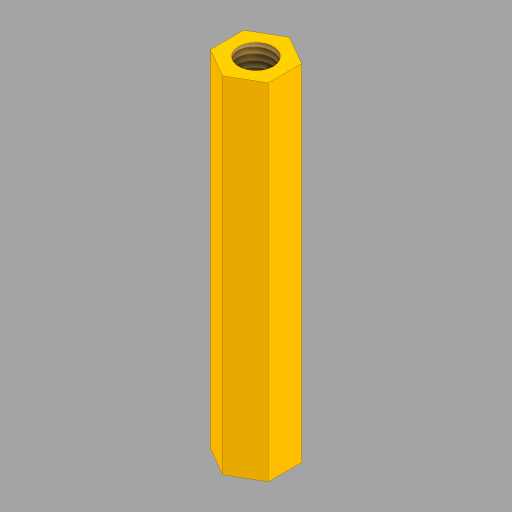
# Autodesk Inventor part: stoyka_40mm
Saved by Autodesk Inventor 2024.2 (Build 282272000, 272)
## iProperties
Created: 2024-01-02
Part Number: stoyka_40mm
Material: Типовые
Document SubType Name: Modeling
Designer: Fedor Orlov
Density: 1 g/cm^3
Appearance: По умолчанию
Author: Fedor Orlov
Autodesk Inventor part; units mm, degrees
ref_plane "YZ Plane" through (0, 0, 0) normal (1, 0, 0) x (0, 1, 0)
ref_plane "XZ Plane" through (0, 0, 0) normal (0, 1, 0) x (-1, 0, 0)
ref_plane "XY Plane" through (0, 0, 0) normal (0, 0, 1) x (1, 0, 0)
sketch "Эскиз1" plane through (0, 0, 0) normal (0, 1, 0) x (-1, 0, 0)
  line L0 (3.35, 1.9341) -> (3.35, -1.9341)
  line L1 (3.35, -1.9341) -> (0, -3.8682)
  line L2 (0, -3.8682) -> (-3.35, -1.9341)
  line L3 (-3.35, -1.9341) -> (-3.35, 1.9341)
  line L4 (-3.35, 1.9341) -> (0, 3.8682)
  line L5 (0, 3.8682) -> (3.35, 1.9341)
  circle A0 centre (0, 0) radius 2
  dimension "d0" = 6.7
  dimension "d1" = 6.7
  dimension "d2" = 4
  constraints: 12 end point, 2 coincident, 1 centre point, 13 other
  measures "d0" distance between parallel lines of L1 L4
  measures "d1" horizontal distance of L0.end L3.end
  measures "d2" diameter of A0
extrude "Выдавливание1" add sketch "Эскиз1" along normal blind 40
thread "Резьба1" size "M4x0.7" class "6H" standard "ANSI Metric M Profile" full length
equation "\"d0\" = d1"
